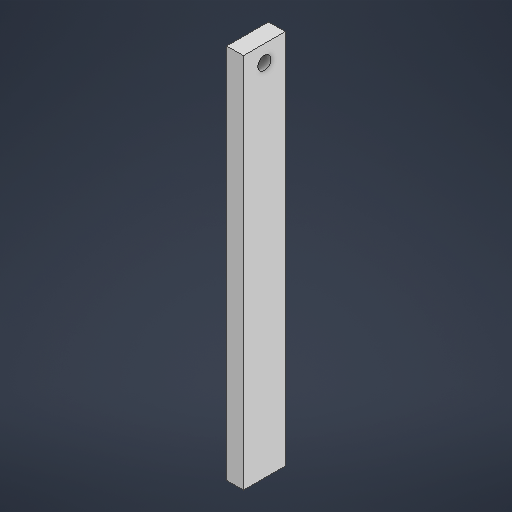
# Autodesk Inventor part: Apoio
Saved by Autodesk Inventor 2026.2 (Build 302298000, 298)
## iProperties
Created: 2026-02-25
Part Number: Apoio
Material: Genérico
Document SubType Name: Modeling
Designer: Ian
Density: 1 g/cm^3
Appearance: Padrão
Author: Ian
Autodesk Inventor part; units mm, degrees
ref_plane "YZ Plane" through (0, 0, 0) normal (1, 0, 0) x (0, 1, 0)
ref_plane "XZ Plane" through (0, 0, 0) normal (0, 1, 0) x (-1, 0, 0)
ref_plane "XY Plane" through (0, 0, 0) normal (0, 0, 1) x (1, 0, 0)
sketch "Esboço1" plane through (0, 0, 0) normal (0, 1, 0) x (-1, 0, 0)
  line L0 (-10, 25) -> (10, 25)
  line L1 (10, 25) -> (10, -25)
  line L2 (10, -25) -> (-10, -25)
  line L3 (-10, -25) -> (-10, 25)
  line L4 (-10, 25) -> (10, -25) construction
  line L5 (10, 25) -> (-10, -25) construction
  point P0 (0, 0)
  dimension "d0" = 20
  dimension "d1" = 50
  constraints: 12 end point, 2 midpoint, 2 parallel, 1 horizontal, 1 perpendicular
  measures "d0" distance of L1.end L2.end
  measures "d1" distance of L0.end L1.end
extrude "Extrusão1" add sketch "Esboço1" along normal blind 450
sketch "Esboço2" plane through (10, 0, 25) normal (1, 0, 0) x (0, 0, -1)
  circle A0 centre (25, 430) radius 8
  line L0 (0, 450) -> (50, 450) projected
  point P0 (25, 0)
  point P1 (25, 450)
  dimension "d4" = 16
  dimension "d7" = 0
  dimension "d8" = 20
  constraints: 1 centre point, 1 midpoint
  measures "d4" diameter of A0
  measures "d7" horizontal distance of point (25, 450) A0.centre
  measures "d8" distance from line of L0 A0.centre
extrude "Extrusão2" cut sketch "Esboço2" against normal blind 450
